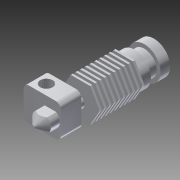
# Autodesk Inventor part: HexagonHotEndBody
Saved by Autodesk Inventor 2015 (Build 190159000, 159)
## iProperties
Created: 2014-10-09
Part Number: HexagonHotEndBody
Material: Aluminum 6061
Document SubType Name: Modeling
Designer: Jack
Density: 2.7 g/cm^3
Appearance: Aluminum - Flat
Author: Jack
Autodesk Inventor part; units mm, degrees
ref_plane "YZ Plane" through (0, 0, 0) normal (1, 0, 0) x (0, 1, 0)
ref_plane "XZ Plane" through (0, 0, 0) normal (0, 1, 0) x (-1, 0, 0)
sketch "Sketch1" plane through (0, 0, 0) normal (0, 1, 0) x (-1, 0, 0)
  line L0 (9.4108, 0) -> (4.7054, -8.15)
  line L1 (4.7054, -8.15) -> (-4.7054, -8.15)
  line L2 (-4.7054, -8.15) -> (-9.4108, 0)
  line L3 (-9.4108, 0) -> (-4.7054, 8.15)
  line L4 (-4.7054, 8.15) -> (4.7054, 8.15)
  line L5 (4.7054, 8.15) -> (9.4108, 0)
  point P0 (0, 0)
  point P1 (0, 0)
  dimension "d0" = 16.3
  constraints: 12 end point, 1 coincident, 1 horizontal, 13 other
  measures "d0" distance between parallel lines of L1 L4
extrude "Extrusion1" add sketch "Sketch1" along normal blind 1
pattern_linear "Rectangular Pattern1" count 10 spacing 2.3 along (0, 1, 0) of "Extrusion1"
sketch "Sketch2" plane through (-4.7054, 21.7, 8.15) normal (0, 1, 0) x (1, 0, 0)
  circle A0 centre (4.7054, 8.15) radius 7.9
  dimension "d6" = 15.8
  constraints: 1 centre point, 1 coincident
  measures "d6" diameter of A0
extrude "Extrusion2" add sketch "Sketch2" along normal blind 4.65
sketch "Sketch3" plane through (0, 26.35, 0) normal (0, 1, 0) x (1, 0, 0)
  circle A0 centre (0, 0) radius 7.9 projected
  circle A1 centre (0, 0) radius 6
  dimension "d9" = 12
  constraints: 1 centre point, 1 coincident
  measures "d9" diameter of A1
extrude "Extrusion3" add sketch "Sketch3" along normal blind 4.65 contours A1
sketch "Sketch4" plane through (0, 31, 0) normal (0, 1, 0) x (1, 0, 0)
  circle A0 centre (0, 0) radius 7.9 projected
extrude "Extrusion4" add sketch "Sketch4" along normal blind 4.67
sketch "Sketch5" plane through (0, 0, 0) normal (0, -1, 0) x (1, 0, 0)
  circle A0 centre (0, 0) radius 3
  dimension "d14" = 6
  constraints: 1 centre point, 1 coincident
  measures "d14" diameter of A0
extrude "Extrusion5" add sketch "Sketch5" against normal up to surface (21.7 mm away)
sketch "Sketch6" plane through (0, 0, 0) normal (0, -1, 0) x (1, 0, 0)
  circle A0 centre (0, 0) radius 1.25
  dimension "d17" = 2.5
  constraints: 1 centre point, 1 coincident
  measures "d17" diameter of A0
extrude "Extrusion6" add sketch "Sketch6" along normal blind 1
sketch "Sketch7" plane through (0, -1, 0) normal (0, -1, 0) x (1, 0, 0)
  circle A0 centre (0, 0) radius 1.25 projected
  circle A1 centre (0, 0) radius 3
  dimension "d20" = 6
  constraints: 1 centre point, 1 coincident
  measures "d20" diameter of A1
extrude "Extrusion7" add sketch "Sketch7" along normal blind 3.5 contours A0 | A1
sketch "Sketch8" plane through (0, -4.5, 0) normal (0, -1, 0) x (1, 0, 0)
  circle A0 centre (0, 0) radius 3 projected
  line L0 (5, 8) -> (-13, 8)
  line L1 (-13, 8) -> (-13, -8)
  line L2 (-13, -8) -> (5, -8)
  line L3 (5, -8) -> (5, 8)
  dimension "d23" = 18
  dimension "d24" = 16
  dimension "d25" = 5
  dimension "d26" = 8
  constraints: 8 end point, 2 parallel, 1 horizontal, 1 perpendicular
  measures "d23" distance of L2.end L1.end
  measures "d24" distance of L1.end L0.end
  measures "d25" distance from line of A0.centre L3
  measures "d26" distance from line of L0 A0.centre
extrude "Extrusion8" add sketch "Sketch8" along normal blind 10 contours A0 | L3 L2 L1 L0
fillet "Fillet1" radius 2.5 4 edges at (5, -9.5, -8) (5, -9.5, 8) (-13, -9.5, 8) (-13, -9.5, -8)
sketch "Sketch9" plane through (0, -14.5, 0) normal (0, -1, 0) x (1, 0, 0)
  circle A0 centre (0, 0) radius 4.5
  dimension "d30" = 9
  constraints: 1 centre point, 1 coincident
  measures "d30" diameter of A0
extrude "Extrusion9" add sketch "Sketch9" along normal blind 4.4
ref_plane "Work Plane1" through (0, -22.8, 0) normal (0, -1, 0) x (1, 0, 0)
sketch "Sketch10" plane through (0, -22.8, 0) normal (0, -1, 0) x (1, 0, 0)
  circle A0 centre (0, 0) radius 0.6
  dimension "d34" = 1.2
  constraints: 1 centre point, 1 coincident
  measures "d34" diameter of A0
loft "Loft1" add profiles "Sketch10" section 2 edges at (-4.5, -18.9, 0)
sketch "Sketch11" plane through (0, -14.5, 0) normal (0, -1, 0) x (1, 0, 0)
  circle A0 centre (0, 0) radius 4.5 projected
  line L0 (-2.8284, -3.5) -> (2.8284, -3.5)
  line L1 (-2.8284, 3.5) -> (2.8284, 3.5)
  dimension "d39" = 7
  dimension "d40" = 3.5
  constraints: 4 end point, 4 point on circle, 1 horizontal, 1 parallel
  measures "d39" distance between parallel lines of L0 L1
  measures "d40" distance from line of A0.centre L0
extrude "Extrusion10" cut sketch "Sketch11" along normal blind 6.4 contours L1 A0 | A0 L0
sketch "Sketch12" plane through (0, -22.8, 0) normal (0, -1, 0) x (1, 0, 0)
  circle A0 centre (0, 0) radius 0.6 projected
  circle A1 centre (0, 0) radius 0.2
  dimension "d43" = 0.4
  constraints: 1 centre point, 1 coincident
  measures "d43" diameter of A1
extrude "Extrusion11" cut sketch "Sketch12" against normal up to surface (8.3 mm away) contours A1
sketch "Sketch13" plane through (0, 35.67, 0) normal (0, 1, 0) x (1, 0, 0)
  circle A0 centre (0, 0) radius 0.2 projected
  circle A1 centre (0, 0) radius 3.07
  dimension "d46" = 6.14
  constraints: 1 centre point, 1 coincident
  measures "d46" diameter of A1
extrude "Extrusion12" cut sketch "Sketch13" against normal up to surface (9.32 mm away) contours A0 | A1
sketch "Sketch14" plane through (0, 26.35, 0) normal (0, 1, 0) x (1, 0, 0)
  circle A0 centre (0, 0) radius 3 projected
  circle A1 centre (0, 0) radius 1
  dimension "d49" = 2
  constraints: 1 centre point, 1 coincident
  measures "d49" diameter of A1
extrude "Extrusion13" cut sketch "Sketch14" against normal up to surface (40.85 mm away) contours A1
sketch "Sketch16" plane through (2.5, -4.5, -8) normal (0, 0, -1) x (-1, 0, 0)
  line L0 (13, 0) -> (0, 0) projected
  line L1 (15.5, -10) -> (15.5, 0) projected
  circle A0 centre (9.5, -5) radius 3
  point P0 (2.5, 4.5)
  dimension "d57" = 6
  dimension "d58" = 5
  dimension "d59" = 6
  constraints: 1 centre point
  measures "d57" diameter of A0
  measures "d58" distance from line of L0 A0.centre
  measures "d59" distance from line of L1 A0.centre
extrude "Extrusion15" cut sketch "Sketch16" against normal up to next
sketch "Sketch17" plane through (2.5, -4.5, -8) normal (0, 0, -1) x (-1, 0, 0)
  circle A0 centre (9.5, -5) radius 3 projected
  line L0 (13, 0) -> (0, 0) projected
  circle A1 centre (2.5, -5) radius 1.5
  point P0 (2.5, 4.5)
  dimension "d62" = 3
  dimension "d63" = 7
  dimension "d64" = 5
  constraints: 1 centre point
  measures "d62" diameter of A1
  measures "d63" distance of A0.centre A1.centre
  measures "d64" distance from line of L0 A1.centre
extrude "Extrusion16" cut sketch "Sketch17" against normal blind 5 contours A1
body "Solid1"
